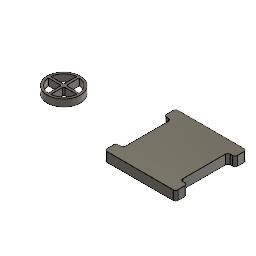
DKVprogetto_1.2 v1 (Autodesk Fusion 360 design; units mm, degrees)
Autodesk Fusion 360 part; units mm, degrees
sketch "Sketch1" plane through (0, 0, 0) normal (0, 1, 0) x (1, 0, 0)
  line L0 (-40, -10) -> (100, -10)
  line L1 (-40, 140) -> (100, 140)
  line L2 (-45, -5) -> (-45, 10)
  line L3 (-45, 135) -> (-45, 120)
  line L4 (-40, 15) -> (-35, 15)
  line L5 (-30, 20) -> (-30, 110)
  line L6 (100, 15) -> (95, 15)
  line L7 (90, 20) -> (90, 110)
  line L8 (-40, 115) -> (-35, 115)
  line L9 (-45, 120) -> (-45, 135)
  line L10 (105, 135) -> (105, 120)
  line L11 (100, 115) -> (95, 115)
  line L12 (-45, -5) -> (-45, 10)
  line L13 (105, -5) -> (105, 10)
  line L14 (25, 140) -> (25, -10)
  line L15 (-30, 65) -> (90, 65)
  arc A0 (-40, 15) -> (-45, 10) centre (-40, 10) ccw
  arc A1 (-35, 15) -> (-30, 20) centre (-35, 20) ccw
  arc A2 (-45, -5) -> (-40, -10) centre (-40, -5) ccw
  arc A3 (90, 20) -> (95, 15) centre (95, 20) ccw
  arc A4 (105, 10) -> (100, 15) centre (100, 10) ccw
  arc A5 (100, -10) -> (105, -5) centre (100, -5) ccw
  arc A6 (95, 115) -> (90, 110) centre (95, 110) ccw
  arc A7 (100, 115) -> (105, 120) centre (100, 120) ccw
  arc A8 (105, 135) -> (100, 140) centre (100, 135) ccw
  arc A9 (-40, 140) -> (-45, 135) centre (-40, 135) ccw
  arc A10 (-45, 120) -> (-40, 115) centre (-40, 120) ccw
  arc A11 (-30, 110) -> (-35, 115) centre (-35, 110) ccw
  circle A12 centre (-210, 70) radius 35
  line L16 (-210, 70) -> (-210, 67.5)
  line L17 (-210, 70) -> (-210, 72.5)
  line L18 (-215, 72.5) -> (-239.8957, 72.5)
  line L19 (-205, 72.5) -> (-180.1043, 72.5)
  line L20 (-205, 67.5) -> (-180.1043, 67.5)
  line L21 (-207.5, 65) -> (-207.5, 40.1043)
  line L22 (-212.5, 75) -> (-212.5, 99.8957)
  line L23 (-215, 67.5) -> (-239.8957, 67.5)
  arc A13 (-212.5, 65) -> (-215, 67.5) centre (-215, 65) ccw
  line L24 (-212.5, 65) -> (-212.5, 40.1043)
  arc A14 (-215, 72.5) -> (-212.5, 75) centre (-215, 75) ccw
  arc A15 (-207.5, 75) -> (-205, 72.5) centre (-205, 75) ccw
  line L25 (-207.5, 75) -> (-207.5, 99.8957)
  arc A16 (-205, 67.5) -> (-207.5, 65) centre (-205, 65) ccw
  arc A17 (-207.5, 40.1043) -> (-180.1043, 67.5) centre (-210, 70) ccw
  arc A18 (-239.8957, 67.5) -> (-212.5, 40.1043) centre (-210, 70) ccw
  arc A19 (-180.1043, 72.5) -> (-207.5, 99.8957) centre (-210, 70) ccw
  arc A20 (-212.5, 99.8957) -> (-239.8957, 72.5) centre (-210, 70) ccw
  dimension "d9" = 70
  dimension "d12" = 2.5
  dimension "d13" = 2.5
  measures "d9" diameter of A12
extrude "Extrude1" add sketch "Sketch1" along normal blind 15 makes body 1 at (10, 0, -80) makes body 2 at (-175.1739, 10, -66.5151)
extrude "Extrude2" add 1 faces at (10, 15, -80) along direction (0, 1, 0) blind 5 on bodies 1 bodies 1
